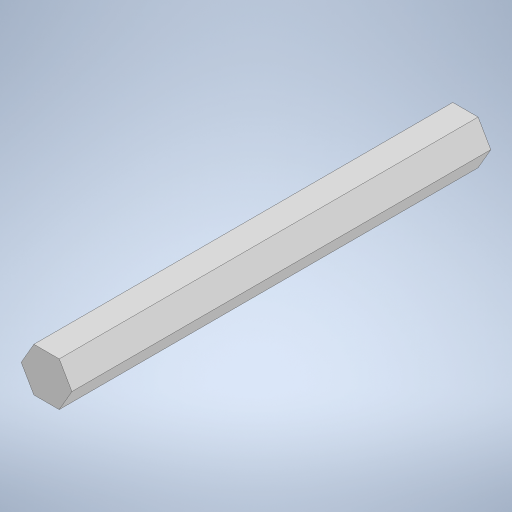
# Autodesk Inventor part: hex shaft
Saved by Autodesk Inventor 2023 (Build 270158000, 158)
## iProperties
Created: 2022-12-01
Part Number: hex shaft
Material: Generic
Document SubType Name: Modeling
Designer: victo
Density: 1 g/cm^3
Appearance: Default
Author: victo
Autodesk Inventor part; units mm, degrees
ref_plane "YZ Plane" through (0, 0, 0) normal (1, 0, 0) x (0, 1, 0)
ref_plane "XZ Plane" through (0, 0, 0) normal (0, 1, 0) x (-1, 0, 0)
ref_plane "XY Plane" through (0, 0, 0) normal (0, 0, 1) x (1, 0, 0)
sketch "Sketch1" plane through (0, 0, 0) normal (0, 0, 1) x (1, 0, 0)
  line L0 (-4.3602, -2.3462) -> (5.1648, -2.3462)
  line L1 (5.1648, -2.3462) -> (9.9273, -10.5951)
  line L2 (9.9273, -10.5951) -> (5.1648, -18.844)
  line L3 (5.1648, -18.844) -> (-4.3602, -18.844)
  line L4 (-4.3602, -18.844) -> (-9.1227, -10.5951)
  line L5 (-9.1227, -10.5951) -> (-4.3602, -2.3462)
  point P0 (0, 0)
  dimension "d0" = 9.525
  dimension "d1" = 9.525
  dimension "d2" = 9.525
  dimension "d3" = 9.525
  dimension "d4" = 9.525
  dimension "d6" = 9.525
  dimension "d7" = 120
  dimension "d8" = 120
  dimension "d9" = 120
  dimension "d10" = 120
  dimension "d11" = 120
  constraints: 12 end point, 1 horizontal
  measures "d0" distance of L0.start L0.end
  measures "d1" distance of L0.end L1.end
  measures "d2" distance of L1.end L2.end
  measures "d3" distance of L2.end L3.end
  measures "d4" distance of L3.end L4.end
  measures "d6" distance of L4.end L5.end
  measures "d7" angle of L1 L0
  measures "d8" angle of L2 L1
  measures "d9" angle of L2 L3
  measures "d10" angle of L3 L4
  measures "d11" angle of L5 L4
extrude "Extrusion1" add sketch "Sketch1" along normal blind 157.48
body "Solid1"
